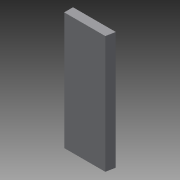
# Autodesk Inventor part: toprectangle
Saved by Autodesk Inventor 2015 (Build 190159000, 159)
## iProperties
Created: 2015-02-03
Part Number: toprectangle
Material: Generic
Document SubType Name: Modeling
Designer: rubidium
Density: 1 g/cm^3
Appearance: Default
Author: rubidium
Autodesk Inventor part; units mm, degrees
ref_plane "YZ Plane" through (0, 0, 0) normal (1, 0, 0) x (0, 1, 0)
ref_plane "XZ Plane" through (0, 0, 0) normal (0, 1, 0) x (-1, 0, 0)
ref_plane "XY Plane" through (0, 0, 0) normal (0, 0, 1) x (1, 0, 0)
sketch "Sketch1" plane through (0, 0, 0) normal (0, 1, 0) x (-1, 0, 0)
  line L0 (88.9, 0) -> (0, 0)
  line L1 (0, 0) -> (0, -19.05)
  line L2 (0, -19.05) -> (88.9, -19.05)
  line L3 (88.9, -19.05) -> (88.9, 0)
  line L4 (0, 0) -> (-3.6409, -19.05)
  line L5 (-3.6409, -19.05) -> (0, -19.05)
  line L6 (-3.6409, -19.05) -> (0, -19.05)
  dimension "d0" = 88.9
  dimension "d1" = 19.05
  dimension "d4" = 100.82
  constraints: 14 end point, 3 equal length, 2 horizontal, 1 coincident, 1 perpendicular
  measures "d0" distance of L0.start L0.end
  measures "d1" distance of L0.end L1.end
  measures "d4" angle of L0 L4
extrude "Extrusion1" add sketch "Sketch1" along normal blind 254
body "Solid1"
